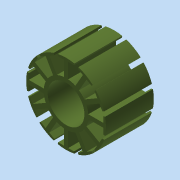
# Autodesk Inventor part: Stator
Saved by Autodesk Inventor 2015 (Build 190159000, 159)
## iProperties
Created: 2015-12-24
Part Number: Stator
Material: Steel, Mild, Welded
Document SubType Name: Modeling
Designer: Raphael
Density: 7.85 g/cm^3
Appearance: Olive Green
stator_length: 1.181 in
stator_id: 0.906 in
Author: Raphael
Autodesk Inventor part; units mm, degrees
ref_plane "YZ Plane" through (0, 0, 0) normal (1, 0, 0) x (0, 1, 0)
ref_plane "XZ Plane" through (0, 0, 0) normal (0, 1, 0) x (-1, 0, 0)
ref_plane "XY Plane" through (0, 0, 0) normal (0, 0, 1) x (1, 0, 0)
sketch "Sketch1" plane through (0, 0, 0) normal (0, 0, 1) x (1, 0, 0)
  circle A0 centre (0, 0) radius 11.5
  circle A1 centre (0, 0) radius 25
  line L0 (-1.315, 13.9381) -> (-1.315, 23.3542)
  line L1 (-1.315, 23.3542) -> (-4.9641, 23.3542)
  line L2 (-4.9641, 23.3542) -> (-5.1978, 24.4537)
  line L3 (1.315, 13.9381) -> (1.315, 23.3542)
  line L4 (1.315, 23.3542) -> (4.9641, 23.3542)
  line L5 (4.9641, 23.3542) -> (5.1978, 24.4537)
  arc A2 (5.1978, 24.4537) -> (-5.1978, 24.4537) centre (0, 0) ccw
  circle A3 centre (0, 0) radius 14
  line L6 (-8.1079, 11.4133) -> (-12.8159, 19.5679)
  line L7 (-12.8159, 19.5679) -> (-15.9762, 17.7433)
  line L8 (-15.9762, 17.7433) -> (-16.7283, 18.5786)
  line L9 (-5.8303, 12.7282) -> (-10.5383, 20.8829)
  line L10 (-10.5383, 20.8829) -> (-7.3781, 22.7074)
  line L11 (-7.3781, 22.7074) -> (-7.7254, 23.7764)
  arc A4 (-7.7254, 23.7764) -> (-16.7283, 18.5786) centre (0, 0) ccw
  line L12 (-12.7282, 5.8303) -> (-20.8829, 10.5383)
  line L13 (-20.8829, 10.5383) -> (-22.7074, 7.3781)
  line L14 (-22.7074, 7.3781) -> (-23.7764, 7.7254)
  line L15 (-11.4133, 8.1079) -> (-19.5679, 12.8159)
  line L16 (-19.5679, 12.8159) -> (-17.7433, 15.9762)
  line L17 (-17.7433, 15.9762) -> (-18.5786, 16.7283)
  arc A5 (-18.5786, 16.7283) -> (-23.7764, 7.7254) centre (0, 0) ccw
  line L18 (-13.9381, -1.315) -> (-23.3542, -1.315)
  line L19 (-23.3542, -1.315) -> (-23.3542, -4.9641)
  line L20 (-23.3542, -4.9641) -> (-24.4537, -5.1978)
  line L21 (-13.9381, 1.315) -> (-23.3542, 1.315)
  line L22 (-23.3542, 1.315) -> (-23.3542, 4.9641)
  line L23 (-23.3542, 4.9641) -> (-24.4537, 5.1978)
  arc A6 (-24.4537, 5.1978) -> (-24.4537, -5.1978) centre (0, 0) ccw
  line L24 (-11.4133, -8.1079) -> (-19.5679, -12.8159)
  line L25 (-19.5679, -12.8159) -> (-17.7433, -15.9762)
  line L26 (-17.7433, -15.9762) -> (-18.5786, -16.7283)
  line L27 (-12.7282, -5.8303) -> (-20.8829, -10.5383)
  line L28 (-20.8829, -10.5383) -> (-22.7074, -7.3781)
  line L29 (-22.7074, -7.3781) -> (-23.7764, -7.7254)
  arc A7 (-23.7764, -7.7254) -> (-18.5786, -16.7283) centre (0, 0) ccw
  line L30 (-5.8303, -12.7282) -> (-10.5383, -20.8829)
  line L31 (-10.5383, -20.8829) -> (-7.3781, -22.7074)
  line L32 (-7.3781, -22.7074) -> (-7.7254, -23.7764)
  line L33 (-8.1079, -11.4133) -> (-12.8159, -19.5679)
  line L34 (-12.8159, -19.5679) -> (-15.9762, -17.7433)
  line L35 (-15.9762, -17.7433) -> (-16.7283, -18.5786)
  arc A8 (-16.7283, -18.5786) -> (-7.7254, -23.7764) centre (0, 0) ccw
  line L36 (1.315, -13.9381) -> (1.315, -23.3542)
  line L37 (1.315, -23.3542) -> (4.9641, -23.3542)
  line L38 (4.9641, -23.3542) -> (5.1978, -24.4537)
  line L39 (-1.315, -13.9381) -> (-1.315, -23.3542)
  line L40 (-1.315, -23.3542) -> (-4.9641, -23.3542)
  line L41 (-4.9641, -23.3542) -> (-5.1978, -24.4537)
  arc A9 (-5.1978, -24.4537) -> (5.1978, -24.4537) centre (0, 0) ccw
  line L42 (8.1079, -11.4133) -> (12.8159, -19.5679)
  line L43 (12.8159, -19.5679) -> (15.9762, -17.7433)
  line L44 (15.9762, -17.7433) -> (16.7283, -18.5786)
  line L45 (5.8303, -12.7282) -> (10.5383, -20.8829)
  line L46 (10.5383, -20.8829) -> (7.3781, -22.7074)
  line L47 (7.3781, -22.7074) -> (7.7254, -23.7764)
  arc A10 (7.7254, -23.7764) -> (16.7283, -18.5786) centre (0, 0) ccw
  line L48 (12.7282, -5.8303) -> (20.8829, -10.5383)
  line L49 (20.8829, -10.5383) -> (22.7074, -7.3781)
  line L50 (22.7074, -7.3781) -> (23.7764, -7.7254)
  line L51 (11.4133, -8.1079) -> (19.5679, -12.8159)
  line L52 (19.5679, -12.8159) -> (17.7433, -15.9762)
  line L53 (17.7433, -15.9762) -> (18.5786, -16.7283)
  arc A11 (18.5786, -16.7283) -> (23.7764, -7.7254) centre (0, 0) ccw
  line L54 (13.9381, 1.315) -> (23.3542, 1.315)
  line L55 (23.3542, 1.315) -> (23.3542, 4.9641)
  line L56 (23.3542, 4.9641) -> (24.4537, 5.1978)
  line L57 (13.9381, -1.315) -> (23.3542, -1.315)
  line L58 (23.3542, -1.315) -> (23.3542, -4.9641)
  line L59 (23.3542, -4.9641) -> (24.4537, -5.1978)
  arc A12 (24.4537, -5.1978) -> (24.4537, 5.1978) centre (0, 0) ccw
  line L60 (11.4133, 8.1079) -> (19.5679, 12.8159)
  line L61 (19.5679, 12.8159) -> (17.7433, 15.9762)
  line L62 (17.7433, 15.9762) -> (18.5786, 16.7283)
  line L63 (12.7282, 5.8303) -> (20.8829, 10.5383)
  line L64 (20.8829, 10.5383) -> (22.7074, 7.3781)
  line L65 (22.7074, 7.3781) -> (23.7764, 7.7254)
  arc A13 (23.7764, 7.7254) -> (18.5786, 16.7283) centre (0, 0) ccw
  line L66 (5.8303, 12.7282) -> (10.5383, 20.8829)
  line L67 (10.5383, 20.8829) -> (7.3781, 22.7074)
  line L68 (7.3781, 22.7074) -> (7.7254, 23.7764)
  line L69 (8.1079, 11.4133) -> (12.8159, 19.5679)
  line L70 (12.8159, 19.5679) -> (15.9762, 17.7433)
  line L71 (15.9762, 17.7433) -> (16.7283, 18.5786)
  arc A14 (16.7283, 18.5786) -> (7.7254, 23.7764) centre (0, 0) ccw
  dimension "d1" = 50
  dimension "d0" = 23
  dimension "d2" = 24
  dimension "d3" = 28
  dimension "d6" = 360
  constraints: 144 end point, 26 point on circle, 14 centre point, 4 coincident, 2 equal length, 2 perpendicular, 1 collinear, 1 vertical, 198 other
  measures "d0" diameter of A0
  measures "d2" angle of L5 L2
  measures "d3" diameter of A3
extrude "Extrusion1" add sketch "Sketch1" along normal blind 30 contours A3 | L5 L4 L3 A3 L0 L1 L2 A1
pattern_circular "Circular Pattern1" count 12 over 360 about axis through (0, 0, -10) along (0, 0, 1) of "Extrusion1"
equation "\"d1\" = stator_diameter"
equation "\"d0\" = stator_id"
equation "\"d8\" = stator_length"
equation "\"stator_length\" = 30"
equation "\"stator_id\" = 23"
equation "\"stator_diameter\" = 50"
body "Solid1"
